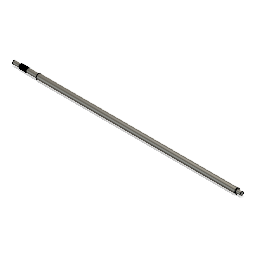
Linear Assembly (Autodesk Fusion 360 archive; units mm, degrees)
design "SFU1204"
Autodesk Fusion 360 part; units mm, degrees
sketch "Sketch1" plane through (0, 0, 0) normal (0, 0, 1) x (1, 0, 0)
  line L0 (0, 0) -> (0, 4)
  line L1 (0, 4) -> (15, 4)
  line L2 (15, 4) -> (15, 4.5)
  line L3 (15, 4.5) -> (31, 4.5)
  line L4 (31, 4.5) -> (31, 5)
  line L5 (31, 5) -> (54, 5)
  line L6 (489, 6) -> (489, 4)
  line L7 (489, 4) -> (499, 4)
  line L8 (499, 4) -> (499, 0)
  line L9 (499, 0) -> (0, 0)
  line L10 (54, 5) -> (54, 6)
  line L11 (54, 6) -> (489, 6)
  dimension "d1" = 4
  dimension "d2" = 15
  dimension "d3" = 4.5
  dimension "d4" = 5
  dimension "d5" = 4
  dimension "d8" = 6
  dimension "d9" = 10
  dimension "d12" = 435
  dimension "d13" = 31
  dimension "d14" = 54
  constraint coincident L0.start L9.end
  constraint vertical L0
  constraint perpendicular L0 L1
  constraint perpendicular L1 L2
  constraint perpendicular L2 L3
  constraint perpendicular L3 L4
  constraint perpendicular L4 L5
  constraint perpendicular L5 L6
  constraint perpendicular L6 L7
  constraint perpendicular L7 L8
  constraint horizontal L9
  constraint perpendicular L5 L10
  constraint horizontal L11
  measures "d1" distance of L0.start L0.end
  measures "d2" distance of L0.end L1.end
  measures "d3" distance of L3 L9
  measures "d4" distance of L5 L9
  measures "d5" distance of L7 L9
  measures "d8" distance of L9 L11
  measures "d9" distance of L6 L8
  measures "d12" distance of L6 L10
  measures "d13" distance of L0 L4
  measures "d14" distance of L0 L10
revolve "Revolve1" add sketch "Sketch1" angle 360 about axis through (499, 0, 0) along (-1, 0, 0)
thread "Thread1" "ISO Metric profile 10.0 M10x1.5 6g" major diameter 9.85 minor diameter 8.141 pitch 1.5 angle 60 modelled right hand crest width 0.1875 on face at (25.6667, 4.4944, 0.2243) crest through (14.9062, 4.925, 0)
